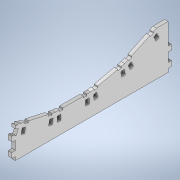
# Autodesk Inventor part: switchplate-support-06-ext
Saved by Autodesk Inventor 2020 (Build 240168000, 168)
## iProperties
Created: 2019-06-27
Material: Acier, galvanisé
Document SubType Name: Modeling
Designer: Thibault
Density: 7.85 g/cm^3
Appearance: Anodisé - Bronze foncé subtil
Mass: 11.7255 g
Surface Area: 33.7109 cm^2
Volume: 1.4937 cm^3
Part Number: switchplate-support-06-ext
sa_0: 0.400 nd
height_shift: 0,000 mm
base_height: 25,000 mm
switchplate_depth: 111,000 mm
Author: Thibault
Autodesk Inventor part; units mm, degrees
ref_plane "YZ Plane" through (0, 0, 0) normal (1, 0, 0) x (0, 1, 0)
ref_plane "XZ Plane" through (0, 0, 0) normal (0, 1, 0) x (-1, 0, 0)
ref_plane "XY Plane" through (0, 0, 0) normal (0, 0, 1) x (1, 0, 0)
sketch "Anchor (to extra support)" plane through (0, 0, 0) normal (0, 0, 1) x (1, 0, 0)
  line L0 (12.7767, 14.8837) -> (14.7767, 14.8837)
  line L1 (14.7767, 14.8837) -> (14.7767, 11.8837)
  line L2 (14.7767, 11.8837) -> (12.7767, 11.8837)
  line L3 (12.7767, 11.8837) -> (12.7767, 14.8837)
  point P0 (14.0267, 11.8837)
  dimension "d219" = 2
  dimension "d220" = 3
  measures "d219" distance of L1.end L2.end
  measures "d220" distance of L0.end L1.end
sketch "Unit" plane through (0, 0, 0) normal (0, 0, 1) x (1, 0, 0)
  line L0 (14.375, 16.4474) -> (15.075, 16.4474)
  line L1 (15.075, 16.4474) -> (15.075, 15.6474)
  line L2 (15.075, 15.6474) -> (17.075, 15.6474)
  line L3 (17.075, 15.6474) -> (17.075, 16.4474)
  line L4 (17.075, 16.4474) -> (22.875, 16.4474)
  line L5 (28.675, 16.4474) -> (28.675, 15.6474)
  line L6 (28.675, 15.6474) -> (30.675, 15.6474)
  line L7 (30.675, 15.6474) -> (30.675, 16.4474)
  line L8 (30.675, 16.4474) -> (31.375, 16.4474)
  line L9 (22.875, 19.1721) -> (22.875, 15.8971) construction
  line L10 (22.875, 16.4474) -> (28.675, 16.4474)
  line L11 (13.875, 14.0474) -> (15.875, 14.0474)
  line L12 (15.875, 14.0474) -> (15.875, 11.0474)
  line L13 (15.875, 11.0474) -> (13.875, 11.0474)
  line L14 (13.875, 11.0474) -> (13.875, 14.0474)
  line L15 (29.875, 14.0474) -> (31.875, 14.0474)
  line L16 (31.875, 14.0474) -> (31.875, 11.0474)
  line L17 (31.875, 11.0474) -> (29.875, 11.0474)
  line L18 (29.875, 11.0474) -> (29.875, 14.0474)
  point P0 (20.0288, 26.7181)
  dimension "d4" = 0.8
  dimension "d5" = 2
  dimension "d8" = 11.6
  dimension "d16" = 2
  dimension "d19" = 0.7
  dimension "d123" = 17
  dimension "d258" = 7
  dimension "d259" = 7
  dimension "d260" = 1.6
  measures "d4" distance of L1.start L1.end
  measures "d5" distance of L1.end L2.end
  measures "d8" distance of L5.start L3.end
  measures "d16" distance of L5.end L6.end
  measures "d19" distance of L7.end point (31.375, 16.447)
  measures "d123" distance of point (31.375, 16.447) point (14.375, 16.447)
sketch "Anchor (to main structure)" plane through (0, 0, 0) normal (0, 0, 1) x (1, 0, 0)
  line L0 (0, 0) -> (2, 0)
  line L1 (2, 0) -> (2, 1.75)
  line L2 (2, 0) -> (3, 0) construction
  line L3 (2.25, 2) -> (4.75, 2)
  line L4 (5, 1.75) -> (5, 0)
  line L5 (5, 2) -> (7, 2) construction
  line L6 (10, 0) -> (10, 1.75)
  line L7 (10.25, 2) -> (12.75, 2)
  line L8 (13, 1.75) -> (13, 0)
  line L9 (10, 0) -> (8.35, 0)
  line L10 (8.35, 0) -> (8.35, -2.5)
  line L11 (8.35, -2.5) -> (9.15, -2.5)
  line L12 (9.15, -2.5) -> (9.15, -4.5)
  line L13 (5.85, -4.5) -> (5.85, -2.5)
  line L14 (5.85, -2.5) -> (6.65, -2.5)
  line L15 (6.65, -2.5) -> (6.65, 0)
  line L16 (6.65, 0) -> (5, 0)
  line L17 (13, 0) -> (15, 0)
  line L18 (5.85, -4.5) -> (6.65, -4.5)
  line L19 (9.15, -4.5) -> (8.35, -4.5)
  line L20 (6.65, -4.5) -> (6.65, -6.5)
  line L21 (8.35, -4.5) -> (8.35, -6.5)
  arc A0 (6.65, -6.5) -> (8.35, -6.5) centre (7.5, -6.5) ccw
  arc A1 (2.25, 2) -> (2, 1.75) centre (2.25, 1.75) ccw
  arc A2 (5, 1.75) -> (4.75, 2) centre (4.75, 1.75) ccw
  arc A3 (10.25, 2) -> (10, 1.75) centre (10.25, 1.75) ccw
  arc A4 (13, 1.75) -> (12.75, 2) centre (12.75, 1.75) ccw
  point P0 (9.1321, -0.6227)
  point P1 (2, 2)
  point P2 (10, 2)
  point P3 (13, 2)
  dimension "d2" = 2
  dimension "d71" = 2
  dimension "d73" = 3
  dimension "d74" = 2
  dimension "d76" = 5
  dimension "d79" = 3
  dimension "d80" = 2
  dimension "d102" = 1.65
  dimension "d103" = 2.5
  dimension "d104" = 0.8
  dimension "d105" = 2
  dimension "d114" = 0.8
  dimension "d115" = 1.7
  dimension "d116" = 2.5
  dimension "d117" = 2
  dimension "d170" = 2
  dimension "d171" = 0.8
  dimension "d172" = 0.8
  dimension "d173" = 2
  dimension "d174" = 2
  dimension "d177" = 1.7
  dimension "d178" = 2
  dimension "d218" = 0.25
  measures "d2" distance of point (0, 0) L1.start
  measures "d71" distance of L1.start point (2, 2)
  measures "d73" distance of point (2, 2) L5.start
  measures "d74" distance of L5.start L16.end
  measures "d76" distance of L16.end L9.start
  measures "d79" distance of point (10, 2) point (13, 2)
  measures "d80" distance of point (13, 2) L8.end
  measures "d102" distance of L9.start L9.end
  measures "d103" distance of L9.end L10.end
  measures "d104" distance of L10.end L11.end
  measures "d105" distance of L11.end L12.end
  measures "d114" distance of L13.end L14.end
  measures "d115" distance of L15.end L9.end
  measures "d116" distance of L14.end L15.end
  measures "d117" distance of L9.start point (10, 2)
  measures "d170" distance of L8.end point (15, 0)
  measures "d171" distance of L13.start L18.end
  measures "d172" distance of L12.end L19.end
  measures "d173" distance of L18.end L20.end
  measures "d174" distance of L19.end L21.end
  measures "d177" distance of L18.end L19.end
  measures "d178" distance of L13.start L13.end
  measures "d218" radius of A1
sketch "Sketch1" plane through (0, 0, 0) normal (1, 0, 0) x (0, 1, 0)
  line L0 (0, -111) -> (25, -111)
  line L1 (0, 0) -> (0, -111)
  line L2 (25, 0) -> (0, 0)
  line L3 (25, -111) -> (25, -102.3511)
  line L4 (24.5231, -9.0226) -> (25, -8)
  line L5 (28.2121, -16.9724) -> (22.1003, -16.9724)
  line L6 (24.4083, -9.2688) -> (25, -8)
  line L7 (17.2238, -24.6761) -> (16.6322, -25.9449)
  line L8 (21.9473, -35.6102) -> (15.8356, -35.6102)
  line L9 (16.3291, -27.3117) -> (16.6322, -25.9449)
  line L10 (12.6497, -43.9087) -> (12.3467, -45.2756)
  line L11 (19.8511, -55.1756) -> (13.7394, -55.1756)
  line L12 (12.3467, -46.6756) -> (12.3467, -45.2756)
  line L13 (12.3467, -63.6756) -> (12.3467, -65.0756)
  line L14 (22.0358, -74.7409) -> (15.9241, -74.7409)
  line L15 (12.6497, -66.4424) -> (12.3467, -65.0756)
  line L16 (16.3291, -83.0394) -> (16.6322, -84.4062)
  line L17 (28.3566, -93.3787) -> (22.2449, -93.3787)
  line L18 (17.2238, -85.675) -> (16.6322, -84.4062)
  line L19 (24.4083, -101.0823) -> (25, -102.3511)
  line L20 (25, 0) -> (25, -8)
  line L21 (24.4083, -9.2688) -> (24.1125, -9.9032)
  line L22 (24.1125, -9.9032) -> (23.3875, -9.5652)
  line L23 (23.3875, -9.5652) -> (22.5422, -11.3778)
  line L24 (22.5422, -11.3778) -> (23.2673, -11.7159)
  line L25 (23.2673, -11.7159) -> (20.8161, -16.9724)
  line L26 (18.3649, -22.229) -> (17.6398, -21.8909)
  line L27 (17.6398, -21.8909) -> (16.7946, -23.7036)
  line L28 (16.7946, -23.7036) -> (17.5197, -24.0416)
  line L29 (17.5197, -24.0416) -> (17.2238, -24.6761)
  line L30 (23.2855, -18.1239) -> (20.3173, -16.7399) construction
  line L31 (20.8161, -16.9724) -> (18.3649, -22.229)
  line L32 (22.4445, -7.8014) -> (21.5993, -9.614)
  line L33 (21.5993, -9.614) -> (18.8803, -8.3462)
  line L34 (18.8803, -8.3462) -> (19.7256, -6.5335)
  line L35 (19.7256, -6.5335) -> (22.4445, -7.8014)
  line L36 (15.6826, -22.3023) -> (14.8374, -24.1149)
  line L37 (14.8374, -24.1149) -> (12.1185, -22.8471)
  line L38 (12.1185, -22.8471) -> (12.9637, -21.0345)
  line L39 (12.9637, -21.0345) -> (15.6826, -22.3023)
  line L40 (16.3291, -27.3117) -> (16.1776, -27.9951)
  line L41 (16.1776, -27.9951) -> (15.3966, -27.822)
  line L42 (15.3966, -27.822) -> (14.9637, -29.7746)
  line L43 (14.9637, -29.7746) -> (15.7448, -29.9477)
  line L44 (15.7448, -29.9477) -> (14.4894, -35.6102)
  line L45 (13.2341, -41.2727) -> (12.453, -41.0996)
  line L46 (12.453, -41.0996) -> (12.0201, -43.0522)
  line L47 (12.0201, -43.0522) -> (12.8012, -43.2253)
  line L48 (12.8012, -43.2253) -> (12.6497, -43.9087)
  line L49 (17.1495, -36.2) -> (13.9521, -35.4911) construction
  line L50 (14.4894, -35.6102) -> (13.2341, -41.2727)
  line L51 (14.0943, -26.3041) -> (13.6614, -28.2567)
  line L52 (13.6614, -28.2567) -> (10.7325, -27.6074)
  line L53 (10.7325, -27.6074) -> (11.1654, -25.6548)
  line L54 (11.1654, -25.6548) -> (14.0943, -26.3041)
  line L55 (10.6312, -41.9248) -> (10.1983, -43.8774)
  line L56 (10.1983, -43.8774) -> (7.2695, -43.2281)
  line L57 (7.2695, -43.2281) -> (7.7023, -41.2755)
  line L58 (7.7023, -41.2755) -> (10.6312, -41.9248)
  line L59 (12.3467, -46.6756) -> (12.3467, -47.3756)
  line L60 (12.3467, -47.3756) -> (11.5467, -47.3756)
  line L61 (11.5467, -47.3756) -> (11.5467, -49.3756)
  line L62 (11.5467, -49.3756) -> (12.3467, -49.3756)
  line L63 (12.3467, -49.3756) -> (12.3467, -55.1756)
  line L64 (12.3467, -60.9756) -> (11.5467, -60.9756)
  line L65 (11.5467, -60.9756) -> (11.5467, -62.9756)
  line L66 (11.5467, -62.9756) -> (12.3467, -62.9756)
  line L67 (12.3467, -62.9756) -> (12.3467, -63.6756)
  line L68 (15.0713, -55.1756) -> (11.7963, -55.1756) construction
  line L69 (12.3467, -55.1756) -> (12.3467, -60.9756)
  line L70 (9.9467, -46.1756) -> (9.9467, -48.1756)
  line L71 (9.9467, -48.1756) -> (6.9467, -48.1756)
  line L72 (6.9467, -48.1756) -> (6.9467, -46.1756)
  line L73 (6.9467, -46.1756) -> (9.9467, -46.1756)
  line L74 (9.9467, -62.1756) -> (9.9467, -64.1756)
  line L75 (9.9467, -64.1756) -> (6.9467, -64.1756)
  line L76 (6.9467, -64.1756) -> (6.9467, -62.1756)
  line L77 (6.9467, -62.1756) -> (9.9467, -62.1756)
  line L78 (12.6497, -66.4424) -> (12.8012, -67.1258)
  line L79 (12.8012, -67.1258) -> (12.0201, -67.2989)
  line L80 (12.0201, -67.2989) -> (12.453, -69.2515)
  line L81 (12.453, -69.2515) -> (13.2341, -69.0784)
  line L82 (13.2341, -69.0784) -> (14.4894, -74.7409)
  line L83 (15.7448, -80.4034) -> (14.9637, -80.5766)
  line L84 (14.9637, -80.5766) -> (15.3966, -82.5291)
  line L85 (15.3966, -82.5291) -> (16.1776, -82.356)
  line L86 (16.1776, -82.356) -> (16.3291, -83.0394)
  line L87 (17.1495, -74.1512) -> (13.9521, -74.86) construction
  line L88 (14.4894, -74.7409) -> (15.7448, -80.4034)
  line L89 (10.1983, -66.4737) -> (10.6312, -68.4263)
  line L90 (10.6312, -68.4263) -> (7.7023, -69.0756)
  line L91 (7.7023, -69.0756) -> (7.2695, -67.123)
  line L92 (7.2695, -67.123) -> (10.1983, -66.4737)
  line L93 (13.6614, -82.0944) -> (14.0943, -84.047)
  line L94 (14.0943, -84.047) -> (11.1654, -84.6963)
  line L95 (11.1654, -84.6963) -> (10.7325, -82.7437)
  line L96 (10.7325, -82.7437) -> (13.6614, -82.0944)
  line L97 (17.2238, -85.675) -> (17.5197, -86.3095)
  line L98 (17.5197, -86.3095) -> (16.7946, -86.6476)
  line L99 (16.7946, -86.6476) -> (17.6398, -88.4602)
  line L100 (17.6398, -88.4602) -> (18.3649, -88.1221)
  line L101 (18.3649, -88.1221) -> (20.8161, -93.3787)
  line L102 (23.2673, -98.6352) -> (22.5422, -98.9733)
  line L103 (22.5422, -98.9733) -> (23.3875, -100.786)
  line L104 (23.3875, -100.786) -> (24.1125, -100.4479)
  line L105 (24.1125, -100.4479) -> (24.4083, -101.0823)
  line L106 (23.2855, -92.2272) -> (20.3173, -93.6112) construction
  line L107 (20.8161, -93.3787) -> (23.2673, -98.6352)
  line L108 (14.8374, -86.2362) -> (15.6826, -88.0488)
  line L109 (15.6826, -88.0488) -> (12.9637, -89.3166)
  line L110 (12.9637, -89.3166) -> (12.1185, -87.504)
  line L111 (12.1185, -87.504) -> (14.8374, -86.2362)
  line L112 (21.5993, -100.7371) -> (22.4445, -102.5497)
  line L113 (22.4445, -102.5497) -> (19.7256, -103.8176)
  line L114 (19.7256, -103.8176) -> (18.8803, -102.005)
  line L115 (18.8803, -102.005) -> (21.5993, -100.7371)
  point P0 (0, -41.2578)
  point P1 (0, -43.2578)
  point P2 (0, -54.8578)
  point P3 (0, -56.8578)
  dimension "height" = 25
  dimension "d193" = 25
  dimension "k1_angle" = 115
  dimension "k1_a" = 1.4
  dimension "k1_b" = 1.4
  dimension "k2_angle" = 102.5
  dimension "k2_a" = 1.4
  dimension "k2_b" = 1.4
  dimension "k3_angle" = 90
  dimension "k3_a" = 1.4
  dimension "k3_b" = 1.4
  dimension "k4_angle" = 77.5
  dimension "k4_a" = 1.4
  dimension "k4_b" = 1.4
  dimension "k5_angle" = 65
  dimension "k5_a" = 1.4
  dimension "k5_b" = 1.4
  dimension "d257" = 8
  constraints: 42 end point, 12 horizontal, 4 vertical, 1 collinear, 1 vertical alignment, 19 other
  measures "height" distance of L2.start L1.start
  measures "d193" distance of L0.end L0.start
  measures "k1_a" distance of L4.end L6.start
  measures "k1_b" distance of L7.end L7.start
  measures "k2_a" distance of L9.start L7.end
  measures "k2_b" distance of L10.end L10.start
  measures "k3_angle" angle to the sketch y axis of L11
  measures "k3_a" distance of L12.start L10.end
  measures "k3_b" distance of L13.end L13.start
  measures "k4_a" distance of L15.start L13.end
  measures "k4_b" distance of L16.end L16.start
  measures "k5_a" distance of L18.start L16.end
  measures "k5_b" distance of L3.end L19.start
  measures "d257" distance of L2.start L4.end
extrude "Base" add sketch "Sketch1" along normal blind 2
sketch "Sketch2" plane through (0, 0, 0) normal (-1, 0, 0) x (0, 0, 1)
  line L0 (-109, 0) -> (-2, 0)
  line L1 (-179.6233, 19.237) -> (-179.6233, -29.346)
  line L2 (139.5944, 112.9292) -> (139.5944, -29.346)
  line L3 (139.5944, -29.346) -> (-179.6233, -29.346)
  line L4 (-111, 20) -> (-111, 0) construction
  line L5 (-109, 15) -> (-109, 103.8044)
  line L6 (-109, 103.8044) -> (-179.6233, 103.8044)
  line L7 (-179.6233, 103.8044) -> (-179.6233, 19.237)
  line L8 (-2, 15) -> (-2, 112.9292)
  line L9 (-2, 112.9292) -> (139.5944, 112.9292)
  line L10 (0, 25) -> (0, 0) projected
  line L11 (0, 0) -> (-111, 0) projected
  line L12 (0, 25) -> (0, 0) projected
  line L13 (-111, 0) -> (-111, 25) projected
  line L14 (-109, 0) -> (-109, 2)
  line L15 (-109, 2) -> (-110.75, 2)
  line L16 (-109, 2) -> (-109, 3) construction
  line L17 (-111, 2.25) -> (-111, 4.75)
  line L18 (-110.75, 5) -> (-109, 5)
  line L19 (-111, 5) -> (-111, 7) construction
  line L20 (-109, 10) -> (-110.75, 10)
  line L21 (-111, 10.25) -> (-111, 12.75)
  line L22 (-110.75, 13) -> (-109, 13)
  line L23 (-109, 10) -> (-109, 8.35)
  line L24 (-109, 8.35) -> (-106.5, 8.35)
  line L25 (-106.5, 8.35) -> (-106.5, 9.15)
  line L26 (-106.5, 9.15) -> (-104.5, 9.15)
  line L27 (-104.5, 5.85) -> (-106.5, 5.85)
  line L28 (-106.5, 5.85) -> (-106.5, 6.65)
  line L29 (-106.5, 6.65) -> (-109, 6.65)
  line L30 (-109, 6.65) -> (-109, 5)
  line L31 (-109, 13) -> (-109, 15)
  line L32 (-104.5, 5.85) -> (-104.5, 6.65)
  line L33 (-104.5, 9.15) -> (-104.5, 8.35)
  line L34 (-104.5, 6.65) -> (-102.5, 6.65)
  line L35 (-104.5, 8.35) -> (-102.5, 8.35)
  arc A0 (-102.5, 6.65) -> (-102.5, 8.35) centre (-102.5, 7.5) ccw
  arc A1 (-111, 2.25) -> (-110.75, 2) centre (-110.75, 2.25) ccw
  arc A2 (-110.75, 5) -> (-111, 4.75) centre (-110.75, 4.75) ccw
  arc A3 (-111, 10.25) -> (-110.75, 10) centre (-110.75, 10.25) ccw
  arc A4 (-110.75, 13) -> (-111, 12.75) centre (-110.75, 12.75) ccw
  line L36 (-2, 15) -> (-2, 13)
  line L37 (-2, 13) -> (-0.25, 13)
  line L38 (-2, 13) -> (-2, 12) construction
  line L39 (0, 12.75) -> (0, 10.25)
  line L40 (-0.25, 10) -> (-2, 10)
  line L41 (0, 10) -> (0, 8) construction
  line L42 (-2, 5) -> (-0.25, 5)
  line L43 (0, 4.75) -> (0, 2.25)
  line L44 (-0.25, 2) -> (-2, 2)
  line L45 (-2, 5) -> (-2, 6.65)
  line L46 (-2, 6.65) -> (-4.5, 6.65)
  line L47 (-4.5, 6.65) -> (-4.5, 5.85)
  line L48 (-4.5, 5.85) -> (-6.5, 5.85)
  line L49 (-6.5, 9.15) -> (-4.5, 9.15)
  line L50 (-4.5, 9.15) -> (-4.5, 8.35)
  line L51 (-4.5, 8.35) -> (-2, 8.35)
  line L52 (-2, 8.35) -> (-2, 10)
  line L53 (-2, 2) -> (-2, 0)
  line L54 (-6.5, 9.15) -> (-6.5, 8.35)
  line L55 (-6.5, 5.85) -> (-6.5, 6.65)
  line L56 (-6.5, 8.35) -> (-8.5, 8.35)
  line L57 (-6.5, 6.65) -> (-8.5, 6.65)
  arc A5 (-8.5, 8.35) -> (-8.5, 6.65) centre (-8.5, 7.5) ccw
  arc A6 (0, 12.75) -> (-0.25, 13) centre (-0.25, 12.75) ccw
  arc A7 (-0.25, 10) -> (0, 10.25) centre (-0.25, 10.25) ccw
  arc A8 (0, 4.75) -> (-0.25, 5) centre (-0.25, 4.75) ccw
  arc A9 (-0.25, 2) -> (0, 2.25) centre (-0.25, 2.25) ccw
  point P0 (-111, 0)
  point P1 (110, 20)
  point P2 (-2, 0)
  point P3 (0, 20)
  point P4 (-110, 20)
  point P5 (0, 22)
  point P6 (-43.2578, 0)
  point P7 (0, 17.9896)
  point P8 (0, 19.5524)
  point P9 (-110, 14.3891)
  point P10 (0, 35.5246)
  point P11 (-110, 28.3499)
  constraints: 18 end point, 4 horizontal, 4 vertical, 2 parallel, 1 collinear, 1 perpendicular, 1 point on line, 12 other
extrude "Standard anchors" cut sketch "Sketch2" against normal through all
sketch "Esquisse7" plane through (0, 0, 0) normal (-1, 0, 0) x (0, 0, 1)
  line L0 (-104.5, 8.35) -> (-102.5, 8.35) construction
  line L1 (-106.5, 9.15) -> (-104.5, 9.15) construction
  line L2 (-104.5, 5.85) -> (-106.5, 5.85) construction
  line L3 (-102.5, 6.65) -> (-104.5, 6.65) construction
  line L4 (-109, 9.15) -> (-100.5, 9.15)
  line L5 (-109, 5.85) -> (-100.5, 5.85)
  line L6 (-109, 10) -> (-109, 8.35) construction
  line L7 (-109, 9.15) -> (-109, 5.85)
  arc A0 (-102.5, 6.65) -> (-102.5, 8.35) centre (-102.5, 7.5) ccw projected
  line L8 (-100.5, 5.85) -> (-100.5, 9.15)
  point P0 (1.5, 20)
  point P1 (108.5, 20)
  point P2 (108.5, 0)
  point P3 (1.5, 0)
  point P4 (-2, 10)
  point P5 (-2, 5)
  point P6 (7.6691, 10.85)
  point P7 (8.8147, 9.7576)
  point P8 (-108.5, 0)
  point P9 (-102.77, 8.35)
  point P10 (-100.7609, 7.9198)
  dimension "d203" = 2
  constraints: 8 end point, 2 collinear, 1 perpendicular, 1 vertical, 2 other
  measures "d203" distance from line of L8 A0.centre
extrude "No back screw hole" add sketch "Esquisse7" against normal up to surface (2 mm away)
sketch "Esquisse11" plane through (0, 0, 0) normal (-1, 0, 0) x (0, 0, 1)
  line L0 (-13.18, 9.15) -> (-2, 9.15)
  line L1 (-2, 9.15) -> (-2, 5.85)
  line L2 (-2, 5.85) -> (-13.18, 5.85)
  line L3 (-13.18, 5.85) -> (-13.18, 9.15)
  line L4 (-2, 8.35) -> (-2, 10) projected
  line L5 (-6.5, 9.15) -> (-4.5, 9.15) projected
  line L6 (-4.5, 5.85) -> (-6.5, 5.85) projected
  arc A0 (-8.5, 8.35) -> (-8.5, 6.65) centre (-8.5, 7.5) ccw projected
  dimension "d231" = 4.68
  constraints: 8 end point, 3 collinear, 2 parallel, 1 horizontal, 1 perpendicular
  measures "d231" distance from line of L3 A0.centre
extrude "No front screw hole  (normal plate)" [suppressed]
sketch "Esquisse8" plane through (0, 0, 0) normal (-1, 0, 0) x (0, 0, 1)
  line L0 (-111, 0) -> (-109, 0) projected
  line L1 (0, 0) -> (-20.4545, 0)
  line L2 (0, 74.3401) -> (0, 0)
  line L3 (0, 12.75) -> (0, 10.25) projected
  line L4 (-20.4545, 0) -> (-20.4545, 74.3401)
  line L5 (-20.4545, 74.3401) -> (0, 74.3401)
  point P0 (110, 0)
  point P1 (0, 12)
  dimension "d232" = 20.4545
  constraints: 8 end point, 2 collinear, 1 horizontal, 1 parallel, 1 vertical
  measures "d232" distance of L1.start L1.end
extrude "Short plate" cut sketch "Esquisse8" against normal through all
sketch "Esquisse9" plane through (0, 0, 0) normal (-1, 0, 0) x (0, 0, 1)
  line L0 (-109, 0) -> (-111, 0) projected
  line L1 (-20.4545, 0) -> (-20.4545, 20) construction
  line L2 (-22.4545, 15) -> (-22.4545, 25.6415)
  line L3 (-22.4545, 25.6415) -> (0.6033, 25.6415)
  line L4 (0.6033, 25.6415) -> (0.6033, 0)
  line L5 (0.6033, 0) -> (-22.4545, 0)
  line L6 (-2, 0) -> (-109, 0) projected
  line L7 (-22.4545, 15) -> (-22.4545, 13)
  line L8 (-22.4545, 13) -> (-20.7045, 13)
  line L9 (-22.4545, 13) -> (-22.4545, 12) construction
  line L10 (-20.4545, 12.75) -> (-20.4545, 10.25)
  line L11 (-20.7045, 10) -> (-22.4545, 10)
  line L12 (-20.4545, 10) -> (-20.4545, 8) construction
  line L13 (-22.4545, 5) -> (-20.7045, 5)
  line L14 (-20.4545, 4.75) -> (-20.4545, 2.25)
  line L15 (-20.7045, 2) -> (-22.4545, 2)
  line L16 (-22.4545, 5) -> (-22.4545, 6.65)
  line L17 (-22.4545, 6.65) -> (-24.9545, 6.65)
  line L18 (-24.9545, 6.65) -> (-24.9545, 5.85)
  line L19 (-24.9545, 5.85) -> (-26.9545, 5.85)
  line L20 (-26.9545, 9.15) -> (-24.9545, 9.15)
  line L21 (-24.9545, 9.15) -> (-24.9545, 8.35)
  line L22 (-24.9545, 8.35) -> (-22.4545, 8.35)
  line L23 (-22.4545, 8.35) -> (-22.4545, 10)
  line L24 (-22.4545, 2) -> (-22.4545, 0)
  line L25 (-26.9545, 9.15) -> (-26.9545, 8.35)
  line L26 (-26.9545, 5.85) -> (-26.9545, 6.65)
  line L27 (-26.9545, 8.35) -> (-28.9545, 8.35)
  line L28 (-26.9545, 6.65) -> (-28.9545, 6.65)
  arc A0 (-28.9545, 8.35) -> (-28.9545, 6.65) centre (-28.9545, 7.5) ccw
  arc A1 (-20.4545, 12.75) -> (-20.7045, 13) centre (-20.7045, 12.75) ccw
  arc A2 (-20.7045, 10) -> (-20.4545, 10.25) centre (-20.7045, 10.25) ccw
  arc A3 (-20.4545, 4.75) -> (-20.7045, 5) centre (-20.7045, 4.75) ccw
  arc A4 (-20.7045, 2) -> (-20.4545, 2.25) centre (-20.7045, 2.25) ccw
  point P0 (0, 0)
  point P1 (22.3526, 0)
  point P2 (22.3526, 15.0824)
  point P3 (-22.3526, 15.0824)
  point P4 (-20.4545, 12.2831)
  point P5 (-20.4545, 20)
  constraints: 8 end point, 2 horizontal, 1 collinear, 1 perpendicular, 1 vertical, 3 other
extrude "Front anchor (short plate)" cut sketch "Esquisse9" against normal through all
sketch "Sketch6" plane through (0, 0, 0) normal (-1, 0, 0) x (0, 0, 1)
  line L0 (-22.4545, 9.15) -> (-29.9545, 9.15)
  line L1 (-29.9545, 9.15) -> (-29.9545, 5.85)
  line L2 (-29.9545, 5.85) -> (-22.4545, 5.85)
  line L3 (-22.4545, 5.85) -> (-22.4545, 9.15)
  line L4 (-26.9545, 9.15) -> (-24.9545, 9.15) projected
  line L5 (-24.9545, 5.85) -> (-26.9545, 5.85) projected
  line L6 (-22.4545, 8.35) -> (-22.4545, 10) projected
  arc A0 (-28.9545, 8.35) -> (-28.9545, 6.65) centre (-28.9545, 7.5) ccw projected
  dimension "d253" = 1
  constraints: 8 end point, 3 collinear, 2 parallel, 1 horizontal, 1 perpendicular
  measures "d253" distance from line of L1 A0.centre
extrude "No front screw hole  (short plate)" add sketch "Sketch6" against normal up to surface (2 mm away)
equation "\"d16\" = d5"
equation "\"d19\" = d18"
equation "\"depth_shift\" = 2"
equation "\"angle\" = 12.5deg"
equation "\"a_default\" = 1.4"
equation "\"b_default\" = 1.4"
equation "\"d18\" = 0.7"
